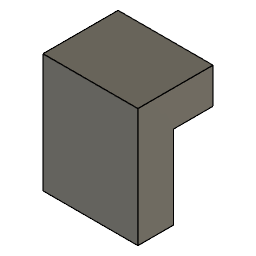
Canal - blocker v3 (Autodesk Fusion 360 design; units mm, degrees)
Autodesk Fusion 360 part; units mm, degrees
sketch "Esquisse1" plane through (0, 0, 0) normal (0, 0, 1) x (1, 0, 0)
  line L0 (21.2537, 17.2704) -> (26.0537, 17.2704)
  line L1 (26.0537, 17.2704) -> (26.0537, 15.4704)
  line L2 (26.0537, 15.4704) -> (21.2537, 15.4704)
  line L3 (21.2537, 15.4704) -> (21.2537, 17.2704)
  dimension "d1" = 4.8
  dimension "d2" = 1.8
  constraint horizontal L0
  constraint vertical L1
  constraint horizontal L2
  constraint vertical L3
  measures "d1" distance of L1 L3
  measures "d2" distance of L0 L2
extrude "Extrusion1" add sketch "Esquisse1" along normal blind 6
sketch "Esquisse2" plane through (0, 17.2704, 0) normal (0, 1, 0) x (-1, 0, 0)
  line L0 (-26.0537, 0) -> (-21.2537, 0)
  line L1 (-21.2537, 0) -> (-21.2537, 6)
  line L2 (-21.2537, 6) -> (-26.0537, 6)
  line L3 (-26.0537, 6) -> (-26.0537, 0)
  line L4 (-21.2537, 6) -> (-26.0537, 6)
  line L5 (-26.0537, 6) -> (-26.0537, 4.2)
  line L6 (-26.0537, 4.2) -> (-21.2537, 4.2)
  line L7 (-21.2537, 4.2) -> (-21.2537, 6)
  dimension "d5" = 1.8
  constraint horizontal L4
  constraint vertical L5
  constraint horizontal L6
  constraint vertical L7
  constraint coincident L3 L5.end
  constraint coincident L1.end L2.start
  measures "d5" distance of L4 L6
extrude "Extrusion2" add sketch "Esquisse2" along normal blind 2 contours L1 L2 L3 L4 L5 L6 L7
